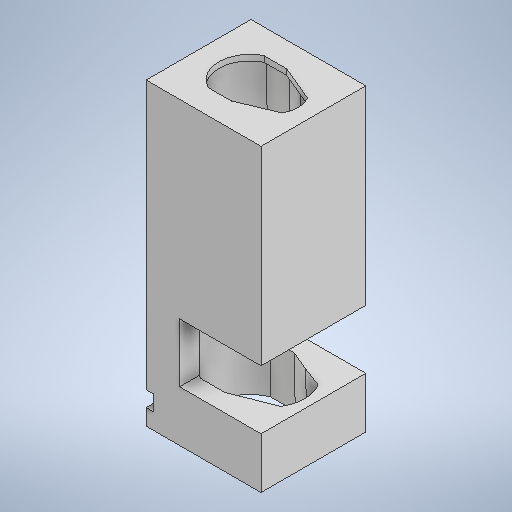
# Autodesk Inventor part: PipetteSleeve
Saved by Autodesk Inventor 2025.1 (Build 291241000, 241)
## iProperties
Created: 2025-01-27
Part Number: PipetteSleeve
Material: Generic
Document SubType Name: Modeling
Designer: 13156
Density: 1 g/cm^3
Appearance: Default
Author: 13156
Autodesk Inventor part; units mm, degrees
ref_plane "YZ Plane" through (0, 0, 0) normal (1, 0, 0) x (0, 1, 0)
ref_plane "XZ Plane" through (0, 0, 0) normal (0, 1, 0) x (-1, 0, 0)
ref_plane "XY Plane" through (0, 0, 0) normal (0, 0, 1) x (1, 0, 0)
sketch "Sketch1" plane through (0, 0, 0) normal (0, 1, 0) x (-1, 0, 0)
  arc A0 (8.935, -11.5681) -> (8.935, 13.0319) centre (3.9712, 0.7319) ccw
  line L0 (8.935, 13.0319) -> (0.335, 13.0319)
  line L1 (8.935, -11.5681) -> (0.335, -11.5681)
  line L2 (0.335, 13.0319) -> (-6.465, 10.2319)
  line L3 (0.335, -11.5681) -> (-6.465, -8.7681)
  line L4 (-6.465, 10.2319) -> (-13.565, 7.5319)
  line L5 (-6.465, -8.7681) -> (-13.565, -6.0681)
  arc A1 (-13.565, 7.5319) -> (-13.565, -6.0681) centre (-3.005, 0.7319) ccw
  line L6 (21.9588, 18.7319) -> (-18.0412, 18.7319)
  line L7 (-18.0412, 18.7319) -> (-18.0412, -17.2681)
  line L8 (-18.0412, -17.2681) -> (21.9588, -17.2681)
  line L9 (21.9588, -17.2681) -> (21.9588, 18.7319)
  line L10 (8.935, -11.5681) -> (8.935, 13.0319) construction
  line L11 (-15.9151, 0.7319) -> (22.2552, 0.7319) construction
  line L12 (0.335, -11.5681) -> (0.335, 13.0319) construction
  line L13 (-13.565, -6.0681) -> (-13.565, 8.8819) construction
  point P0 (0, 0)
  point P1 (-2.143, -1.3001)
  point P2 (8.935, 0.7319)
  point P3 (17.235, 0.7319)
  point P4 (-15.565, 0.7319)
  point P5 (0.335, 0.7319)
  dimension "d0" = 0
  dimension "d1" = 8.6
  dimension "d2" = 8.6
  dimension "d3" = 2.8
  dimension "d4" = 2.8
  dimension "d5" = 6.8
  dimension "d6" = 6.8
  dimension "d7" = 24.6
  dimension "d8" = 7.1
  dimension "d9" = 7.1
  dimension "d10" = 2.7
  dimension "d11" = 2.7
  dimension "d12" = 2
  dimension "d13" = 36
  dimension "d14" = 40
  dimension "d15" = 32.8
  dimension "d16" = 24.6
  dimension "d64" = 21.9588
  dimension "d65" = 18.7319
  dimension "d66" = 13.0319
  dimension "d67" = 41.305
  constraints: 28 end point, 6 point on circle, 4 horizontal, 2 centre point, 2 parallel, 1 midpoint, 1 perpendicular, 1 point on line, 1 vertical, 1 other
  measures "d0" vertical distance of point (17.235, 0.732) point (8.935, 0.732)
  measures "d1" distance of L0.start L0.end
  measures "d2" distance of L1.start L1.end
  measures "d3" vertical distance of L2.end L0.end
  measures "d4" vertical distance of L3.end L1.end
  measures "d5" horizontal distance of L3.end L1.end
  measures "d6" horizontal distance of L2.end L0.end
  measures "d7" distance of L1.start L0.start
  measures "d8" horizontal distance of L4.end L2.end
  measures "d9" horizontal distance of L5.end L3.end
  measures "d10" vertical distance of L3.end L5.end
  measures "d11" vertical distance of L2.end L4.end
  measures "d12" horizontal distance of L5.end point (-15.565, 0.732)
  measures "d13" distance of L6.end L7.end
  measures "d14" distance of L7.end L8.end
  measures "d15" distance of point (-15.565, 0.732) point (17.235, 0.732)
  measures "d16" distance between parallel lines of L0 L1
  measures "d64" distance from line of point (0, 0) L9
  measures "d65" distance from line of L6 point (0, 0)
  measures "d66" distance from line of point (0, 0) L0
extrude "Extrusion1" add sketch "Sketch1" along normal blind 104.4 draft 1
sketch "Sketch2" plane through (0, 0, 0) normal (0, -1, 0) x (1, 0, 0)
  line L0 (-21.9588, -17.2681) -> (-21.9588, 18.7319) projected
  line L1 (18.0412, -17.2681) -> (-21.9588, -17.2681) projected
  line L2 (-21.9588, 18.7319) -> (18.0412, 18.7319)
  line L3 (18.0412, 18.7319) -> (18.0412, -17.2681)
  line L4 (18.0412, -17.2681) -> (-21.9588, -17.2681)
  line L5 (-21.9588, -17.2681) -> (-21.9588, 18.7319)
  line L6 (-21.9588, 18.7319) -> (-23.7811, 20.5542) projected
  line L7 (19.8635, -19.0904) -> (19.8635, 20.5542) projected
  line L8 (-23.7811, 20.5542) -> (19.8635, 20.5542)
  line L9 (19.8635, 20.5542) -> (19.8635, -19.0904)
  line L10 (19.8635, -19.0904) -> (-23.7811, -19.0904)
  line L11 (-23.7811, -19.0904) -> (-23.7811, 20.5542)
  point P0 (0, 0)
  point P1 (19.8635, 20.5542)
  constraints: 16 end point, 4 parallel, 2 horizontal, 2 perpendicular
extrude "Extrusion2" add sketch "Sketch2" against normal blind 104.4
sketch "Sketch3" plane through (19.8635, 0, 20.5542) normal (1, 0, 0) x (0, 0, -1)
  line L0 (42, 38.2) -> (-1, 38.2)
  line L1 (-1, 38.2) -> (-1, 17.7)
  line L2 (-1, 17.7) -> (42, 17.7)
  line L3 (42, 17.7) -> (42, 38.2)
  line L4 (39.6446, 104.4) -> (0, 104.4) projected
  line L5 (0, 0) -> (0, 104.4) projected
  point P0 (20.5542, 0)
  point P1 (17.836, -13.8464)
  point P2 (-1, 27.95)
  point P3 (0, 38.2)
  point P4 (0, 17.7)
  dimension "d21" = 20.5
  dimension "d23" = 43
  dimension "d25" = 86.7
  dimension "d26" = 1
  constraints: 8 end point, 2 parallel, 1 horizontal, 1 midpoint, 1 perpendicular
  measures "d21" distance of L2.end L0.start
  measures "d23" distance from line of L1.end L3
  measures "d25" distance between parallel lines of L4 L2
  measures "d26" distance from line of L5 point (-1, 27.95)
extrude "Extrusion3" cut sketch "Sketch3" against normal blind 30 contours L3 L2 L5 L0
sketch "Sketch5" plane through (0, 104.4, 0) normal (0, 1, 0) x (1, 0, 0)
  line L0 (-8.5676, 9.7458) -> (-0.6955, 9.7458) construction
  line L1 (-8.5676, 9.7458) -> (-8.5676, -14.0116) construction
  line L2 (-0.6955, 9.7458) -> (-0.6955, -15.3944) construction
  line L3 (5.7941, 7.0736) -> (12.3327, 4.5871) construction
  line L4 (12.3327, 4.5871) -> (12.3327, -12.4444) construction
  line L5 (-21.2529, -0.7319) -> (27.3755, -0.7319) construction
  line L6 (-8.5676, 8.9458) -> (-0.6955, 8.9458)
  line L7 (-0.6955, 8.9458) -> (11.6745, 3.7767)
  arc A0 (11.6745, -5.2405) -> (11.6745, 3.7767) centre (4.2943, -0.7319) ccw
  line L8 (11.6745, -5.2405) -> (-0.6955, -10.4096)
  line L9 (-0.6955, -10.4096) -> (-8.5676, -10.4096)
  arc A1 (-8.5676, 8.9458) -> (-8.5676, -10.4096) centre (-3.8211, -0.7319) ccw
  line L10 (-0.6955, 9.7458) -> (5.7941, 7.0736) projected
  line L11 (-0.6955, -11.2096) -> (-8.5676, -11.2096) projected
  arc A2 (12.3327, -6.0509) -> (12.3327, 4.5871) centre (3.005, -0.7319) ccw projected
  line L12 (-23.7811, 19.0904) -> (19.8635, 19.0904) projected
  line L13 (19.8635, -20.5542) -> (-23.7811, -20.5542) projected
  line L14 (-23.7811, 19.0904) -> (19.8635, 19.0904)
  line L15 (19.8635, 19.0904) -> (19.8635, -20.5542)
  line L16 (19.8635, -20.5542) -> (-23.7811, -20.5542)
  line L17 (-23.7811, -20.5542) -> (-23.7811, 19.0904)
  point P0 (0, 0)
  point P1 (-4.6315, 8.9458)
  point P2 (-4.6315, -11.2096)
  point P3 (12.9427, -0.7319)
  point P4 (13.7427, -0.7319)
  point P5 (19.8635, 19.0904)
  dimension "d46" = 0.299
  dimension "d47" = 0.8
  dimension "d48" = 0.8
  dimension "d49" = 10.779
  dimension "d51" = 8.6484
  dimension "d52" = 0.8
  constraints: 24 end point, 6 point on circle, 4 point on line, 3 perpendicular, 3 vertical, 2 centre point, 2 horizontal, 2 midpoint, 2 parallel, 1 equal length, 1 other
  measures "d46" angle of L10 L7
  measures "d47" distance from line of L0 point (-4.632, 8.946)
  measures "d48" distance from line of point (-4.632, -11.21) L9
  measures "d49" radius of A1
  measures "d51" radius of A0
  measures "d52" distance of point (13.743, -0.732) point (12.943, -0.732)
extrude "Extrusion4" add sketch "Sketch5" against normal blind 2
sketch "Sketch6" plane through (-23.7811, 0, -19.0904) normal (-1, 0, 0) x (0, 0, 1)
  line L0 (39.6446, 5.6) -> (0, 5.6)
  line L1 (0, 5.6) -> (0, 11)
  line L2 (0, 11) -> (39.6446, 11)
  line L3 (39.6446, 11) -> (39.6446, 5.6)
  line L4 (39.6446, 0) -> (39.6446, 104.4) projected
  line L5 (0, 0) -> (0, 104.4) projected
  line L6 (39.6446, 0) -> (0, 0) projected
  point P0 (19.0904, 0)
  point P1 (39.6446, 8.3)
  dimension "d55" = 5.4
  dimension "d56" = 0
  dimension "d57" = 0
  dimension "d58" = 5.6
  constraints: 8 end point, 2 parallel, 1 horizontal, 1 midpoint, 1 perpendicular
  measures "d55" distance between parallel lines of L2 L0
  measures "d56" distance from line of L4 point (39.645, 8.3)
  measures "d57" distance between parallel lines of L5 L1
  measures "d58" distance between parallel lines of L0 L6
extrude "Extrusion5" cut sketch "Sketch6" against normal blind 4.5 contours L0 L1 L2 L3
sketch "Sketch7" plane through (-19.2811, 0, -19.0904) normal (-1, 0, 0) x (0, 0, 1)
  line L0 (0, 0) -> (0, 17.7) projected
  line L1 (0, 11) -> (39.6446, 11) projected
  line L2 (0, 5.6295) -> (3, 5.6295)
  line L3 (3, 5.6295) -> (3, 11)
  line L4 (3, 11) -> (0, 11)
  line L5 (0, 11) -> (0, 5.6295)
  point P0 (19.0904, 0)
  dimension "d61" = 3
  constraints: 8 end point, 2 parallel, 2 point on line, 1 horizontal, 1 perpendicular
  measures "d61" distance between parallel lines of L0 L3
extrude "Extrusion6" cut sketch "Sketch7" against normal blind 10.5
sketch "Sketch8" plane through (0, 0, 0) normal (0, -1, 0) x (1, 0, 0)
  line L0 (-21.7811, -17.5904) -> (18.2189, -17.5904)
  line L1 (18.2189, -17.5904) -> (18.2189, 18.9096)
  line L2 (18.2189, 18.9096) -> (-21.7811, 18.9096)
  line L3 (-21.7811, 18.9096) -> (-21.7811, -17.5904)
  line L4 (-23.7811, -19.0904) -> (19.8635, -19.0904) projected
  line L5 (-23.7811, 20.5542) -> (-23.7811, -19.0904) projected
  line L6 (-23.7811, 20.5542) -> (-23.7811, -19.0904) projected
  line L7 (19.8635, -19.0904) -> (19.8635, 20.5542) projected
  line L8 (-23.7811, -19.0904) -> (19.8635, -19.0904)
  line L9 (19.8635, -19.0904) -> (19.8635, 20.5542)
  line L10 (19.8635, 20.5542) -> (-23.7811, 20.5542)
  line L11 (-23.7811, 20.5542) -> (-23.7811, -19.0904)
  point P0 (0, 0)
  dimension "d68" = 36.5
  dimension "d69" = 40
  dimension "d70" = 1.5
  dimension "d71" = 2
  constraints: 16 end point, 4 parallel, 2 horizontal, 2 perpendicular
  measures "d68" distance of L2.end L0.start
  measures "d69" distance of L0.start L0.end
  measures "d70" distance between parallel lines of L4 L0
  measures "d71" distance between parallel lines of L5 L3
extrude "Extrusion7" cut sketch "Sketch8" against normal blind 126.8375
sketch "Sketch9" plane through (-21.7811, 11, -17.5904) normal (-1, 0, 0) x (0, 0, 1)
  circle A0 centre (17.5904, 24) radius 1.95
  circle A1 centre (17.5904, 58.4) radius 1.95
  line L0 (17.5904, -11) -> (17.5904, 93.4) construction
  line L1 (13.8137, 93.4) -> (22.8309, 93.4) construction
  line L2 (0, 93.4) -> (36.5, 93.4) projected
  line L3 (36.5, -11) -> (0, -11) projected
  dimension "d74" = 3.9
  dimension "d75" = 0
  dimension "d76" = 0
  dimension "d78" = 35
  dimension "d79" = 35
  constraints: 2 centre point, 2 end point, 1 equal radius, 1 point on line, 1 vertical
  measures "d74" diameter of A0
  measures "d75" distance from line of L0 A0.centre
  measures "d76" distance from line of L0 A1.centre
  measures "d78" distance from line of L2 A1.centre
  measures "d79" distance from line of L3 A0.centre
extrude "Extrusion8" cut sketch "Sketch9" against normal blind 14.025
body "Solid1"
